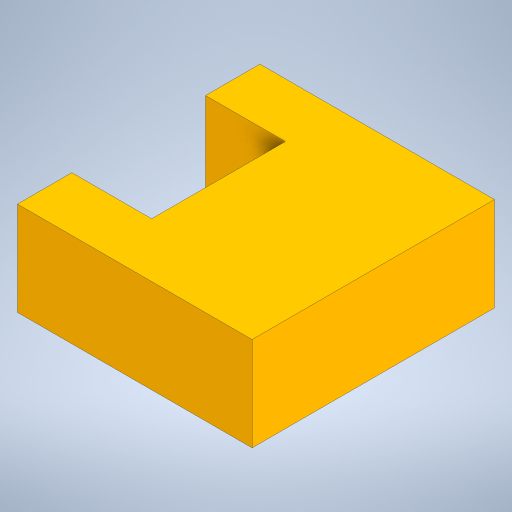
# Autodesk Inventor part: TAPA3
Saved by Autodesk Inventor 2024 (Build 280153000, 153)
## iProperties
Created: 2024-05-01
Part Number: TAPA3
Material: Generic
Document SubType Name: Modeling
Designer: samue
Density: 1 g/cm^3
Appearance: Default
Author: samue
## iProperties of the stored document TAPA3_3DPrint.ipt
Created: 2024-05-01
Part Number: TAPA3_3DPrint
Material: Generic
Document SubType Name: Modeling
Designer: samue
Density: 1 g/cm^3
Appearance: Default
Author: samue
Autodesk Inventor part; units mm, degrees
ref_plane "YZ Plane" through (0, 0, 0) normal (1, 0, 0) x (0, 1, 0)
ref_plane "XZ Plane" through (0, 0, 0) normal (0, 1, 0) x (-1, 0, 0)
ref_plane "XY Plane" through (0, 0, 0) normal (0, 0, 1) x (1, 0, 0)
sketch "Sketch1" plane through (0, 0, 0) normal (0, 1, 0) x (-1, 0, 0)
  line L0 (7.5, 7.75) -> (-7.5, 7.75)
  line L1 (-7.5, 7.75) -> (-7.5, -7.75)
  line L2 (-7.5, -7.75) -> (7.5, -7.75)
  line L3 (7.5, -7.75) -> (7.5, 7.75)
  line L4 (7.5, 7.75) -> (-7.5, -7.75) construction
  line L5 (-7.5, 7.75) -> (7.5, -7.75) construction
  point P0 (0, 0)
  dimension "d0" = 15
  dimension "d1" = 15.5
  constraints: 12 end point, 2 midpoint, 2 parallel, 1 horizontal, 1 perpendicular
  measures "d0" distance of L2.end L1.end
  measures "d1" distance of L1.end L0.end
extrude "Extrusion1" add sketch "Sketch1" along normal blind 6
sketch "Sketch2" plane through (0, 6, 0) normal (0, 1, 0) x (1, 0, 0)
  line L0 (7.5, -7.75) -> (7.5, 7.75) projected
  line L1 (-7.5, 7.75) -> (-7.5, -7.75) projected
  line L2 (-7.5, 4.275) -> (-2.4, 4.275)
  line L3 (-2.4, 4.275) -> (-2.4, -4.275)
  line L4 (-2.4, -4.275) -> (-7.5, -4.275)
  line L5 (-7.5, 0) -> (-2.4, -4.275) construction
  line L6 (-2.4, 4.275) -> (-7.5, 0) construction
  line L7 (-7.5, 4.275) -> (-7.5, -4.275)
  point P0 (0, 0)
  point P1 (-7.5, 0)
  dimension "d4" = 15
  dimension "d5" = 5.1
  dimension "d6" = 8.55
  constraints: 12 end point, 3 midpoint, 1 horizontal, 1 horizontal alignment, 1 parallel, 1 perpendicular
  measures "d4" distance between parallel lines of L0 L1
  measures "d5" distance between parallel lines of L3 L1
  measures "d6" distance between parallel lines of L4 L2
extrude "Extrusion2" cut sketch "Sketch2" against normal blind 8.25
sketch "Sketch3" plane through (-2.4, 6, -4.275) normal (-1, 0, 0) x (0, 0, 1)
  line L0 (0, -1) -> (8.55, -1)
  line L1 (8.55, -1) -> (8.55, -6)
  line L2 (0, -6) -> (0, -1)
  line L3 (0, -1) -> (4.275, -6) construction
  line L4 (8.55, -1) -> (4.275, -6) construction
  line L5 (0, -6) -> (8.55, -6)
  dimension "d9" = 5
  constraints: 12 end point, 2 point on line, 1 horizontal, 1 midpoint, 1 parallel, 1 perpendicular
  measures "d9" distance between parallel lines of L0 L5
extrude "Extrusion3" cut sketch "Sketch3" against normal blind 2
body "Solid1"
